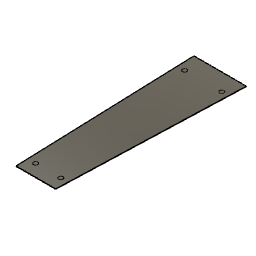
podstawka_bez_karoserii v3 (Autodesk Fusion 360 design; units mm, degrees)
part number: podstawka_bez_karoserii
Autodesk Fusion 360 part; units mm, degrees
sketch "filary_montazowe" plane through (0, 0, 6) normal (0, 0, 1) x (-1, 0, 0)
  circle A0 through (-75.42, -61, -13.4) (-82.29, -57.0336, -13.4) (-82.29, -64.9664, -13.4)
  circle A1 through (-129.5952, -61, -13.4) (-136.4652, -57.0336, -13.4) (-136.4652, -64.9664, -13.4)
  circle A2 through (-129.5952, -61, -13.4) (-136.4652, -57.0336, -13.4) (-136.4652, -64.9664, -13.4)
  circle A3 through (-129.5952, -61, -13.4) (-136.4652, -57.0336, -13.4) (-136.4652, -64.9664, -13.4)
  circle A4 through (-75.42, -61, -13.4) (-82.29, -57.0336, -13.4) (-82.29, -64.9664, -13.4)
  circle A5 through (-129.5952, -61, -13.4) (-136.4652, -57.0336, -13.4) (-136.4652, -64.9664, -13.4)
  circle A6 through (-75.42, -61, -13.4) (-82.29, -57.0336, -13.4) (-82.29, -64.9664, -13.4)
  circle A7 through (-62.68, -395.035, -5.84) (-69.55, -391.0686, -5.84) (-69.55, -399.0014, -5.84)
  circle A8 through (-62.68, -395.035, -5.84) (-69.55, -391.0686, -5.84) (-69.55, -399.0014, -5.84)
  circle A9 through (-142.3352, -395.035, -5.84) (-149.2052, -391.0686, -5.84) (-149.2052, -399.0014, -5.84)
  point P0 (-70, -50)
  point P1 (-70, -384.035)
  dimension "d17" = 9.16
  dimension "d19" = 9.16
  dimension "d21" = 9.16
  dimension "d22" = 9.16
  dimension "d23" = 9.16
  dimension "d24" = 9.16
  dimension "d25" = 9.16
  dimension "d30" = 9.16
  dimension "d31" = 9.16
  dimension "d32" = 9.16
extrude "Extrude1" add sketch "filary_montazowe" along normal blind 15.58 contours A0 A4 A6 | A1 A2 A3 A5 in plane through (0, 0, -7.4) normal (0, 0, 1) makes body 1 at (75.4428, 61.456, -2.2067) makes body 2 at (138.1975, 58.8096, 2.9867)
extrude "Extrude2" add sketch "filary_montazowe" along normal blind 21.54 separate body contours A7 A8 | A9 in plane through (0, 0, 0.16) normal (0, 0, 1) makes body 3 at (71.5638, 396.6015, 14.52) makes body 4 at (143.0071, 392.6468, 14.52)
extrude "Extrude3" cut 2 faces at (66.2574, 396.9061, 21.7) (147.8671, 396.6837, 21.7) along direction (0, 0, -1) blind 18.54 on bodies 3 4 bodies 3 4
extrude "Extrude4" cut 2 faces at (81.178, 61.6476, 8.18) (133.4119, 61.7547, 8.18) along direction (0, 0, -1) blind 10.58 on bodies 1 2 bodies 1 2
extrude "Extrude5" add 2 faces at (81.178, 61.6476, -2.4) (133.4119, 61.7547, -2.4) along direction (0, 0, 1) blind 0.96 on bodies 1 2 bodies 1 2
extrude "Extrude6" add 2 faces at (66.2574, 396.9061, 3.16) (147.8671, 396.6837, 3.16) along direction (0, 0, 1) blind 2.84 on bodies 3 4 bodies 3 4
extrude "Extrude7" add 2 faces at (81.178, 61.6476, -1.44) (133.4119, 61.7547, -1.44) along direction (0, 0, 1) blind 5.84 on bodies 1 2 bodies 1 2
extrude "Extrude8" add 2 faces at (81.178, 61.6476, 4.4) (133.4119, 61.7547, 4.4) along direction (0, 0, 1) blind 1.6 on bodies 1 2 bodies 1 2
sketch "platforma" plane through (0, 0, 6) normal (0, 0, 1) x (1, 0, 0)
  line L0 (50.5279, 431.4967) -> (64.3342, 34.4201)
  line L1 (92.4095, 431.4928) -> (50.5279, 431.4967)
  line L2 (50.528, 431.4929) -> (163.6477, 431.5067)
  line L3 (163.6477, 431.5067) -> (149.841, 34.4197)
  line L4 (92.4095, 431.4928) -> (50.5282, 431.4882)
  line L5 (64.3342, 34.4201) -> (149.841, 34.4197)
  point P0 (80, 61)
  point P1 (134.1752, 61)
  point P2 (146.9152, 395.035)
  point P3 (134.1752, 61)
  point P4 (80, 61)
  point P5 (80, 61)
  point P6 (67.26, 395.035)
  dimension "d53" = 16.58
  dimension "d54" = 16.58
  dimension "d56" = 26.58
  dimension "d57" = 15.455
  dimension "d58" = 15.455
  dimension "d59" = 36.455
  constraint coincident L0 L4.end
  constraint coincident L0 L2.start
  measures "d53" distance of L3 P3
  measures "d54" distance of L0 P5
  measures "d56" distance of P5 L5
  measures "d57" distance of P2 L3
  measures "d58" distance of L0 P6
  measures "d59" distance of L4 P6
extrude "Extrude11" add sketch "platforma" along normal blind 1 separate body contours L0 L1 L2 L3 L4 L5 makes body 5
extrude "Extrude12" cut 2 faces at (81.178, 61.6476, -7.4) (133.4119, 61.7547, -7.4) along direction (0, 0, 1) blind 1.6 on bodies 1 2 bodies 1 2
extrude "Extrude13" cut 2 faces at (66.2574, 396.9061, 0.16) (147.8671, 396.6837, 0.16) along direction (0, 0, 1) blind 2.84 on bodies 3 4 bodies 3 4
cylinder "CylinderPrimitive3" add diameter 6 height 1.6 placed x (0, 1, 0) y (1, 0, 0) z (0, 0, -1) at (80, 61, -5.8) bodies 1
cylinder "CylinderPrimitive4" add diameter 6 height 1.6 placed x (0, 1, 0) y (1, 0, 0) z (0, 0, -1) at (134.1752, 61, -5.8) bodies 2
cylinder "CylinderPrimitive5" add diameter 6.06 height 2.84 placed x (0, 1, 0) y (1, 0, 0) z (0, 0, -1) at (67.26, 395.035, 3) bodies 3
cylinder "CylinderPrimitive6" add diameter 6.06 height 2.84 placed x (0, 1, 0) y (1, 0, 0) z (0, 0, -1) at (146.9152, 395.035, 3) bodies 4
